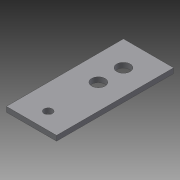
# Autodesk Inventor part: Rail_Pulley_Connector
Saved by Autodesk Inventor 2015 (Build 190159000, 159)
## iProperties
Created: 2017-01-20
Part Number: Rail_Pulley_Connector
Material: Generic
Document SubType Name: Modeling
Designer: Guy
Density: 1 g/cm^3
Appearance: Default
Author: Guy
Autodesk Inventor part; units mm, degrees
ref_plane "YZ Plane" through (0, 0, 0) normal (1, 0, 0) x (0, 1, 0)
ref_plane "XZ Plane" through (0, 0, 0) normal (0, 1, 0) x (-1, 0, 0)
ref_plane "XY Plane" through (0, 0, 0) normal (0, 0, 1) x (1, 0, 0)
sketch "Sketch1" plane through (0, 0, 0) normal (0, 0, 1) x (1, 0, 0)
  line L0 (0, 0) -> (30, 0)
  line L1 (30, 0) -> (30, 70)
  line L2 (30, 70) -> (0, 70)
  line L3 (0, 70) -> (0, 0)
  circle A0 centre (15, 40) radius 4
  circle A1 centre (15, 10) radius 2.5
  circle A2 centre (15, 55) radius 4
  dimension "d0" = 70
  dimension "d1" = 30
  dimension "d2" = 5
  dimension "d3" = 8
  dimension "d5" = 8
  dimension "d6" = 15
  dimension "d7" = 15
  dimension "d9" = 15
  dimension "d10" = 15
  dimension "d13" = 15
  dimension "d14" = 10
  constraints: 8 end point, 3 centre point, 2 parallel, 1 horizontal, 1 perpendicular
  measures "d0" distance of L0.end L1.end
  measures "d1" distance of L1.end L2.end
  measures "d2" diameter of A1
  measures "d3" diameter of A0
  measures "d5" diameter of A2
  measures "d6" distance of A0.centre A2.centre
  measures "d7" distance from line of L3 A1.centre
  measures "d9" distance from line of L3 A2.centre
  measures "d10" distance from line of L3 A0.centre
  measures "d13" distance from line of A2.centre L2
  measures "d14" distance from line of L0 A1.centre
extrude "Extrusion1" add sketch "Sketch1" along normal blind 3
body "Solid1"
